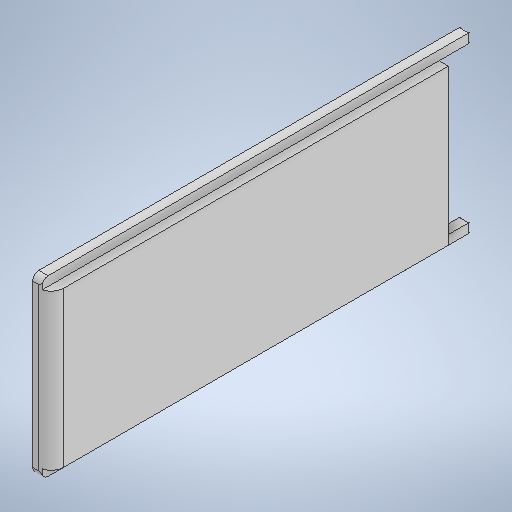
# Autodesk Inventor part: cover
Saved by Autodesk Inventor 2025.4 (Build 294407000, 407)
## iProperties
Created: 2026-03-11
Part Number: cover
Material: Generic
Document SubType Name: Modeling
Designer: Amir
Density: 1 g/cm^3
Appearance: Default
Author: Amir
Autodesk Inventor part; units mm, degrees
ref_plane "YZ Plane" through (0, 0, 0) normal (1, 0, 0) x (0, 1, 0)
ref_plane "XZ Plane" through (0, 0, 0) normal (0, 1, 0) x (-1, 0, 0)
ref_plane "XY Plane" through (0, 0, 0) normal (0, 0, 1) x (1, 0, 0)
sketch "Sketch1" plane through (0, 0, 0) normal (0, 0, 1) x (1, 0, 0)
  line L0 (14.9794, -18.4381) -> (14.9794, 9.5619)
  line L1 (16.4794, -16.9381) -> (17.9794, -16.9381)
  line L2 (17.9794, 8.0619) -> (16.4794, 8.0619)
  line L3 (16.4794, 9.5619) -> (16.4794, 8.0619)
  line L4 (16.4794, -16.9381) -> (16.4794, -18.4381)
  line L5 (14.9794, 9.5619) -> (16.4794, 9.5619)
  line L6 (14.9794, -18.4381) -> (16.4794, -18.4381)
  line L7 (16.4794, -16.9381) -> (14.9794, -16.9381)
  line L8 (16.4794, 8.0619) -> (14.9794, 8.0619)
  line L9 (17.9794, 8.0619) -> (17.9794, -16.9381)
  dimension "d3" = 28
  dimension "d4" = 1.5
  dimension "d5" = 1.5
  dimension "d9" = 1.5
  dimension "d10" = 1.5
  dimension "d11" = 3
  dimension "d12" = 1.5
  dimension "d13" = 1.5
  constraints: 20 end point, 3 parallel, 2 horizontal, 2 point on line, 2 vertical, 1 perpendicular
  measures "d3" distance of L0.start L5.start
  measures "d4" distance between parallel lines of L5 L2
  measures "d5" distance between parallel lines of L1 L6
  measures "d9" distance of L3.end L8.end
  measures "d10" distance between parallel lines of L3 L9
  measures "d11" distance between parallel lines of L0 L9
  measures "d12" distance of L1.start L7.end
  measures "d13" distance of L1.start L1.end
extrude "Extrusion1" add sketch "Sketch1" along normal blind 64
extrude "Extrusion2" add sketch "Sketch1" against normal blind 5 contours L0 L7 L4 L6 | L0 L5 L3 L8
fillet "Fillet1" radius 0.25 8 edges at (15.7294, 9.5619, -5) (16.4794, 8.8119, -5) (15.7294, 8.0619, -5) (14.9794, 8.8119, -5) (16.4794, -17.6881, -5) (15.7294, -16.9381, -5) (14.9794, -17.6881, -5) (15.7294, -18.4381, -5)
fillet "Fillet2" radius 1 2 edges at (15.7294, 9.5619, 64) (15.7294, -18.4381, 64)
fillet "Fillet3" radius 2 1 edges at (17.9794, -4.4381, 64)
body "Solid1"
